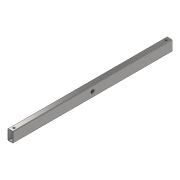
# Autodesk Inventor part: balk
Saved by Autodesk Inventor 2020.3 (Build 243373000, 373)
## iProperties
Created: 2020-09-17
Part Number: balk
Material: Stainless Steel
Document SubType Name: Modeling
Designer: Svend
Density: 8 g/cm^3
Appearance: Semi-Polished
Author: Svend
Autodesk Inventor part; units mm, degrees
ref_plane "YZ Plane" through (0, 0, 0) normal (1, 0, 0) x (0, 1, 0)
ref_plane "XZ Plane" through (0, 0, 0) normal (0, 1, 0) x (-1, 0, 0)
ref_plane "XY Plane" through (0, 0, 0) normal (0, 0, 1) x (1, 0, 0)
sketch "Sketch1" plane through (0, 0, 0) normal (0, 0, 1) x (1, 0, 0)
  line L0 (-7.5, 15) -> (7.5, 15)
  line L1 (7.5, 15) -> (7.5, -15)
  line L2 (7.5, -15) -> (-7.5, -15)
  line L3 (-7.5, -15) -> (-7.5, 15)
  line L4 (-7.5, 15) -> (7.5, -15) construction
  line L5 (7.5, 15) -> (-7.5, -15) construction
  line L6 (-5.5, 13) -> (5.5, 13)
  line L7 (5.5, 13) -> (5.5, -13)
  line L8 (5.5, -13) -> (-5.5, -13)
  line L9 (-5.5, -13) -> (-5.5, 13)
  point P0 (0, 0)
  dimension "d0" = 15
  dimension "d1" = 30
  dimension "d2" = 2
  constraints: 20 end point, 4 parallel, 2 midpoint, 2 perpendicular, 1 horizontal, 3 other
  measures "d0" distance of L1.end L2.end
  measures "d1" distance of L0.end L1.end
  measures "d2" distance between parallel lines of L3 L9
extrude "Extrusion1" add sketch "Sketch1" along normal mid plane 460
sketch "Sketch2" plane through (-7.5, 15, -230) normal (0, 1, 0) x (1, 0, 0)
  circle A0 centre (7.5, -10) radius 3
  circle A1 centre (7.5, -450) radius 3
  line L0 (15, -460) -> (0, -460) projected
  line L1 (0, 0) -> (15, 0) projected
  line L2 (7.5, -450) -> (7.5, -10) construction
  line L3 (0, 0) -> (0, -460) construction
  point P0 (7.5, -230)
  point P1 (7.5, -460)
  point P2 (7.5, 0)
  point P3 (7.5, -230)
  point P4 (0, -230)
  dimension "d5" = 6
  dimension "d6" = 6
  dimension "d7" = 440
  constraints: 3 midpoint, 2 centre point, 2 end point, 2 vertical alignment, 1 horizontal alignment, 1 vertical, 2 other
  measures "d5" diameter of A0
  measures "d6" diameter of A1
  measures "d7" distance of L2.start L2.end
extrude "Extrusion2" cut sketch "Sketch2" against normal through all
sketch "Sketch3" plane through (7.5, -15, -230) normal (1, 0, 0) x (0, 0, -1)
  line L0 (0, 30) -> (0, 0) projected
  line L1 (0, 30) -> (-460, 30) projected
  line L2 (-460, 0) -> (-460, 30) projected
  line L3 (0, 0) -> (-460, 0) projected
  circle A0 centre (-230, 15) radius 5
  point P0 (-230, 30)
  point P1 (0, 15)
  dimension "d10" = 10
  constraints: 2 midpoint, 1 centre point, 1 horizontal alignment, 1 vertical alignment
  measures "d10" diameter of A0
extrude "Extrusion3" cut sketch "Sketch3" against normal through all contours A0
fillet "Fillet1" radius 1 8 edges at (7.5, 15, 0) (-7.5, 15, 0) (7.5, -15, 0) (-7.5, -15, 0) (-5.5, 13, 0) (5.5, 13, 0) (5.5, -13, 0) (-5.5, -13, 0)
body "Solid1"
